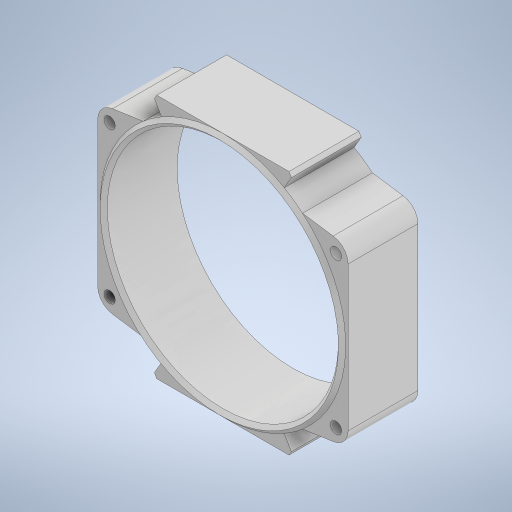
# Autodesk Inventor part: frame_rring3
Saved by Autodesk Inventor 2023.4 (Build 274418000, 418)
## iProperties
Created: 2023-11-26
Part Number: frame_rring3
Material: Generic
Document SubType Name: Modeling
Designer: aaron
Density: 1 g/cm^3
Appearance: Default
Author: aaron
Autodesk Inventor part; units mm, degrees
ref_plane "YZ Plane" through (0, 0, 0) normal (1, 0, 0) x (0, 1, 0)
ref_plane "XZ Plane" through (0, 0, 0) normal (0, 1, 0) x (-1, 0, 0)
ref_plane "XY Plane" through (0, 0, 0) normal (0, 0, 1) x (1, 0, 0)
sketch "Sketch1" plane through (0, 0, 0) normal (0, 0, 1) x (1, 0, 0)
  circle A0 centre (0, 0) radius 48
  arc A1 (-51.7244, -28.0563) -> (-45.7919, -36.955) centre (-44.9997, -30) ccw
  line L0 (-33.0898, -38.808) -> (-45.7919, -36.955)
  arc A2 (-33.0898, -38.808) -> (18.5896, -47.4913) centre (0, 0) ccw
  line L1 (33.7876, -44) -> (18.5896, -47.4913)
  line L2 (54.2078, -44) -> (33.7876, -44)
  line L3 (54.2078, 44) -> (54.2078, -44)
  line L4 (33.7876, 44) -> (54.2078, 44)
  line L5 (18.5896, 47.4913) -> (33.7876, 44)
  arc A3 (18.5896, 47.4913) -> (-33.0898, 38.808) centre (0, 0) ccw
  line L6 (-45.7919, 36.955) -> (-33.0898, 38.808)
  arc A4 (-45.7919, 36.955) -> (-51.7244, 28.0563) centre (-44.9997, 30) ccw
  line L7 (-48.5496, 15.6186) -> (-51.7244, 28.0563)
  arc A5 (-48.5496, 15.6186) -> (-48.5496, -15.6186) centre (0, 0) ccw
  line L8 (-51.7244, -28.0563) -> (-48.5496, -15.6186)
  circle A6 centre (-44.9997, 30) radius 2.875
  circle A7 centre (44.9997, -30) radius 2.875
  circle A8 centre (44.9997, 30) radius 2.875
  circle A9 centre (-44.9997, -30) radius 2.875
  line L9 (64, 42) -> (64, -42)
  line L10 (62, 44) -> (64, 42)
  line L11 (64, -42) -> (62, -44)
  line L12 (61.7922, 44) -> (54.2078, 44)
  line L13 (62, -44) -> (54.2078, -44)
  line L14 (61.7922, 44) -> (62, 44)
  point P0 (61.7922, -44)
  constraints: 30 end point, 10 centre point, 10 point on circle, 2 horizontal, 1 parallel
extrude "Extrusion1" add sketch "Sketch1" along normal blind 29
sketch "Sketch2" plane through (0, 0, 29) normal (0, 0, 1) x (1, 0, 0)
  circle A0 centre (0, 0) radius 51
  circle A1 centre (0, 0) radius 48 projected
  dimension "d2" = 102
  constraints: 1 centre point, 1 coincident
  measures "d2" diameter of A0
extrude "Extrusion2" add sketch "Sketch2" along normal blind 1.5
chamfer "Chamfer1" distance 1.5 angle 45 2 edges at (-51, 0, 30.5) (-48, 0, 30.5)
sketch "Sketch3" plane through (0, 0, 0) normal (0, 0, -1) x (-1, 0, 0)
  circle A0 centre (44.9997, 30) radius 2.875 projected
  circle A1 centre (-44.9997, 30) radius 2.875 projected
  circle A2 centre (-44.9997, -30) radius 2.875 projected
  circle A3 centre (44.9997, -30) radius 2.875 projected
  point P0 (0, 0)
extrude "Extrusion3" add sketch "Sketch3" against normal up to surface (29 mm away)
sketch "Sketch4" plane through (0, 0, 0) normal (0, 0, -1) x (-1, 0, 0)
  circle A0 centre (47.0107, 31.3407) radius 1.6
  circle A1 centre (47.0107, -31.3407) radius 1.6
  circle A2 centre (-47.0107, -31.3407) radius 1.6
  circle A3 centre (-47.0107, 31.3407) radius 1.6
  circle A4 centre (-58, 38) radius 3.025
  line L0 (0, 0) -> (-12.9135, 0)
  circle A5 centre (-58, -38) radius 3.025
  constraints: 6 centre point, 2 end point, 1 horizontal, 1 symmetric about line, 1 other
extrude "Extrusion4" cut sketch "Sketch4" against normal through all
sketch "Sketch5" plane through (0, 0, 29) normal (0, 0, 1) x (1, 0, 0)
  circle A0 centre (-47.0107, -31.3407) radius 1.6 projected
  circle A1 centre (-47.0107, -31.3407) radius 2.35
  circle A2 centre (-47.0107, 31.3407) radius 1.6 projected
  circle A3 centre (-47.0107, 31.3407) radius 2.35
  circle A4 centre (47.0107, 31.3407) radius 1.6 projected
  circle A5 centre (47.0107, 31.3407) radius 2.35
  circle A6 centre (47.0107, -31.3407) radius 1.6 projected
  circle A7 centre (47.0107, -31.3407) radius 2.35
  point P0 (0, 0)
  dimension "d13" = 4.7
  dimension "d14" = 4.7
  dimension "d15" = 4.7
  dimension "d16" = 4.7
  constraints: 4 centre point, 4 coincident
  measures "d13" diameter of A1
  measures "d14" diameter of A3
  measures "d15" diameter of A5
  measures "d16" diameter of A7
extrude "Extrusion5" cut sketch "Sketch5" against normal blind 10.1 contours A0 | A1 | A3 | A5 | A7
sketch "Sketch6" plane through (0, 0, 0) normal (0, 0, -1) x (-1, 0, 0)
  circle A0 centre (47.0107, 31.3407) radius 1.6 projected
  circle A1 centre (47.0107, -31.3407) radius 1.6 projected
  circle A2 centre (-47.0107, -31.3407) radius 1.6 projected
  circle A3 centre (-47.0107, 31.3407) radius 1.6 projected
  point P0 (0, 0)
extrude "Extrusion6" add sketch "Sketch6" against normal blind 15
sketch "Sketch7" plane through (0, 0, 0) normal (0, 0, -1) x (-1, 0, 0)
  circle A0 centre (-44.9997, -30) radius 2.875
  circle A1 centre (-44.9997, 30) radius 2.875
  circle A2 centre (44.9997, 30) radius 2.875
  circle A3 centre (44.9997, -30) radius 2.875
  point P0 (0, 0)
  point P1 (0, 0)
  constraints: 4 centre point
extrude "Extrusion7" cut sketch "Sketch7" against normal blind 14
chamfer "Chamfer2" distance 2.6 angle 45 4 edges at (-42.1247, 30, 14) (-42.1247, -30, 14) (47.8747, -30, 14) (47.8747, 30, 14)
sketch "Sketch8" plane through (33.7876, -44, 0) normal (0, -1, 0) x (1, 0, 0)
  circle A0 centre (23.2124, 14.5) radius 2.875
  line L0 (30.2124, 0) -> (30.2124, 29) projected
  line L1 (0, 0) -> (28.2124, 0) projected
  point P0 (-33.7876, 0)
  dimension "d26" = 5.75
  dimension "d27" = 7
  dimension "d35" = 14.5
  dimension "d60" = 29
  constraints: 1 centre point
  measures "d26" diameter of A0
  measures "d27" distance from line of L0 A0.centre
  measures "d35" distance from line of L1 A0.centre
  measures "d60" distance of L0.start L0.end
extrude "Extrusion8" cut sketch "Sketch8" against normal blind 20
sketch "Sketch11" plane through (0, 0, 0) normal (0, 0, -1) x (-1, 0, 0)
  circle A0 centre (-44.9997, -30) radius 2.875
  circle A1 centre (44.9997, -30) radius 2.875
  circle A2 centre (-44.9997, 30) radius 2.875
  circle A3 centre (44.9997, 30) radius 2.875
  line L0 (-64, 42) -> (-62, 44)
  line L1 (-64, 42) -> (-64, -42)
  line L2 (-62, -44) -> (-64, -42)
  line L3 (-62, -44) -> (-33.7876, -44)
  line L4 (-18.5896, -47.4913) -> (-33.7876, -44)
  arc A4 (-18.5896, -47.4913) -> (33.0898, -38.808) centre (0, 0) ccw
  line L5 (45.7919, -36.955) -> (33.0898, -38.808)
  arc A5 (45.7919, -36.955) -> (51.9997, -30) centre (44.9997, -30) ccw
  line L6 (51.9997, -30) -> (51.9997, 30)
  arc A6 (51.9997, 30) -> (45.7919, 36.955) centre (44.9997, 30) ccw
  line L7 (33.0898, 38.808) -> (45.7919, 36.955)
  arc A7 (33.0898, 38.808) -> (-18.5896, 47.4913) centre (0, 0) ccw
  line L8 (-33.7876, 44) -> (-18.5896, 47.4913)
  line L9 (-33.7876, 44) -> (-62, 44)
  circle A8 centre (0, 0) radius 48
  circle A9 centre (-44.9997, -30) radius 2.875 projected
  circle A10 centre (44.9997, -30) radius 2.875 projected
  circle A11 centre (-44.9997, 30) radius 2.875 projected
  circle A12 centre (44.9997, 30) radius 2.875 projected
  circle A13 centre (-58, 38) radius 3.025 projected
  line L10 (-62, -44) -> (-64, -42) projected
  line L11 (-33.7876, -44) -> (-62, -44) projected
  line L12 (-18.5896, -47.4913) -> (-33.7876, -44) projected
  arc A14 (-18.5896, -47.4913) -> (33.0898, -38.808) centre (0, 0) ccw projected
  line L13 (45.7919, -36.955) -> (33.0898, -38.808) projected
  arc A15 (45.7919, -36.955) -> (51.7244, -28.0563) centre (44.9997, -30) ccw projected
  line L14 (48.5496, -15.6186) -> (51.7244, -28.0563) projected
  arc A16 (48.5496, -15.6186) -> (48.5496, 15.6186) centre (0, 0) ccw projected
  line L15 (51.7244, 28.0563) -> (48.5496, 15.6186) projected
  arc A17 (51.7244, 28.0563) -> (45.7919, 36.955) centre (44.9997, 30) ccw projected
  line L16 (33.0898, 38.808) -> (45.7919, 36.955) projected
  arc A18 (33.0898, 38.808) -> (-18.5896, 47.4913) centre (0, 0) ccw projected
  line L17 (-33.7876, 44) -> (-18.5896, 47.4913) projected
  line L18 (-62, 44) -> (-33.7876, 44) projected
  line L19 (-64, 42) -> (-62, 44) projected
  line L20 (-64, -42) -> (-64, 42) projected
  circle A19 centre (0, 0) radius 48 projected
  constraints: 20 end point, 9 centre point, 8 point on circle
extrude "Extrusion11" add sketch "Sketch11" against normal blind 2 contours L6 A15 L14 A16 L15 A17
sketch "Sketch12" plane through (33.7876, 44, 0) normal (0, 1, 0) x (1, 0, 0)
  circle A0 centre (23.2124, -14.5) radius 2.875 projected
  point P0 (-33.7876, 0)
extrude "Extrusion12" cut sketch "Sketch12" against normal blind 15
sketch "Sketch13" plane through (0, 0, 0) normal (0, 0, -1) x (-1, 0, 0)
  circle A0 centre (-58, 38) radius 3.025 projected
  circle A1 centre (-58, -38) radius 3.025 projected
  point P0 (0, 0)
extrude "Extrusion13" add sketch "Sketch13" against normal blind 20
sketch "Sketch14" plane through (0, 0, 0) normal (0, 0, -1) x (-1, 0, 0)
  circle A0 centre (-58, -38) radius 3.025 projected
  circle A1 centre (-58, 38) radius 3.025 projected
  circle A2 centre (-58, 38) radius 2.875
  circle A3 centre (-58, -38) radius 3.025 projected
  circle A4 centre (-58, -38) radius 2.875
  point P0 (0, 0)
  dimension "d83" = 5.75
  dimension "d84" = 5.75
  constraints: 2 centre point, 2 coincident
  measures "d83" diameter of A2
  measures "d84" diameter of A4
extrude "Extrusion14" cut sketch "Sketch14" against normal blind 10 contours A2 | A4
sketch "Sketch19" plane through (33.7876, 44, 0) normal (0, 1, 0) x (1, 0, 0)
  circle A0 centre (23.2124, -14.5) radius 2.875 projected
  point P0 (-33.7876, 0)
extrude "Extrusion17" cut sketch "Sketch19" against normal blind 15
sketch "Sketch20" plane through (33.7876, -44, 0) normal (0, -1, 0) x (1, 0, 0)
  circle A0 centre (23.2124, 14.5) radius 2.875 projected
  point P0 (-33.7876, 0)
extrude "Extrusion18" cut sketch "Sketch20" against normal blind 15
sketch "Sketch23" plane through (0, 0, 2) normal (0, 0, 1) x (1, 0, 0)
  arc A0 (-51.7244, -28.0563) -> (-51.9997, -30) centre (-44.9997, -30) ccw projected
  line L0 (-48.5496, -15.6186) -> (-51.7244, -28.0563) projected
  arc A1 (-48.5496, 15.6186) -> (-48.5496, -15.6186) centre (0, 0) ccw projected
  line L1 (-51.7244, 28.0563) -> (-48.5496, 15.6186) projected
  arc A2 (-51.9997, 30) -> (-51.7244, 28.0563) centre (-44.9997, 30) ccw projected
  line L2 (-51.9997, 30) -> (-51.9997, -30) projected
extrude "Extrusion19" add sketch "Sketch23" along normal up to surface (27 mm away)
sketch "Sketch24" plane through (0, 0, 0) normal (0, 0, -1) x (-1, 0, 0)
  line L0 (0, 72.608) -> (-70.302, 72.608)
  line L1 (-70.302, 72.608) -> (-70.302, -73.3987)
  line L2 (-70.302, -73.3987) -> (0, -73.3987)
  line L3 (0, -73.3987) -> (0, 72.608)
  point P0 (0, 0)
  constraints: 8 end point, 2 parallel, 1 horizontal, 1 perpendicular
extrude "Extrusion20" cut sketch "Sketch24" against normal through all
mirror "Mirror1" about plane through (0, 72.608, 0) normal (1, 0, 0)
sketch "Sketch25" plane through (0, 0, 0) normal (0, 0, -1) x (-1, 0, 0)
  arc A0 (-33.0898, -38.808) -> (33.0898, -38.808) centre (0, 0) ccw projected
  line L0 (45.7919, -36.955) -> (33.0898, -38.808) projected
  arc A1 (45.7919, -36.955) -> (51.9997, -30) centre (44.9997, -30) ccw projected
  line L1 (51.9997, -30) -> (51.9997, 30) projected
  arc A2 (51.9997, 30) -> (45.7919, 36.955) centre (44.9997, 30) ccw projected
  line L2 (33.0898, 38.808) -> (45.7919, 36.955) projected
  arc A3 (33.0898, 38.808) -> (-33.0898, 38.808) centre (0, 0) ccw projected
  line L3 (-33.0898, 38.808) -> (-45.7919, 36.955) projected
  arc A4 (-45.7919, 36.955) -> (-51.9997, 30) centre (-44.9997, 30) ccw projected
  line L4 (-51.9997, -30) -> (-51.9997, 30) projected
  arc A5 (-51.9997, -30) -> (-45.7919, -36.955) centre (-44.9997, -30) ccw projected
  line L5 (-45.7919, -36.955) -> (-33.0898, -38.808) projected
  circle A6 centre (-44.9997, -30) radius 2.875 projected
  circle A7 centre (-44.9997, 30) radius 2.875 projected
  circle A8 centre (0, 0) radius 48 projected
  circle A9 centre (44.9997, 30) radius 2.875 projected
  circle A10 centre (44.9997, -30) radius 2.875 projected
  line L6 (50.222, 51) -> (-59.2285, 51)
  line L7 (0, 0) -> (39.4707, 68.3652)
  line L8 (0, 0) -> (-39.5796, 68.5538)
  line L9 (0, 0) -> (0, 75.2057)
  line L10 (0, 0) -> (19.7353, 0)
  line L11 (50.222, -51) -> (-59.2285, -51)
  line L12 (0, 0) -> (39.4707, -68.3652)
  line L13 (0, 0) -> (-39.5796, -68.5538)
  point P0 (-29.4449, 51)
  point P1 (-25.5, 44.1673)
  point P2 (0, 51)
  point P3 (25.5, 44.1673)
  point P4 (29.4449, 51)
  point P5 (0, -51)
  point P6 (29.4449, -51)
  point P7 (25.5, -44.1673)
  point P8 (-25.5, -44.1673)
  point P9 (-29.4449, -51)
  dimension "d98" = 30
  dimension "d99" = 30
  constraints: 16 end point, 4 symmetric about line, 2 horizontal, 1 tangent, 1 vertical
  measures "d98" angle of L7 L9
  measures "d99" angle of L8 L9
extrude "Extrusion21" add sketch "Sketch25" against normal up to surface (29 mm away) contours A0 L11 L13 | A0 L12 L11 | L8 L6 A3 | L6 L7 A3
chamfer "Chamfer4" distance 2 angle 45 4 edges at (29.4449, -51, 14.5) (29.4449, 51, 14.5) (-29.4449, 51, 14.5) (-29.4449, -51, 14.5)
equation "\"d35\" = 0.5 * d60"
body "Solid1"
